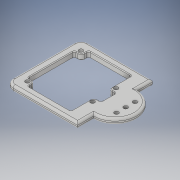
# Autodesk Inventor part: PixyCamMount
Saved by Autodesk Inventor 2018 (Build 220112000, 112)
## iProperties
Created: 2018-09-25
Part Number: PixyCamMount
Material: Generic
Document SubType Name: Modeling
Designer: Jack
Density: 1 g/cm^3
Appearance: Default
Author: Jack
Autodesk Inventor part; units mm, degrees
ref_plane "YZ Plane" through (0, 0, 0) normal (1, 0, 0) x (0, 1, 0)
sketch "Sketch1" plane through (0, 0, 0) normal (0, 1, 0) x (-1, 0, 0)
  line L0 (0, 0) -> (57.15, 0)
  line L1 (63.5, -6.35) -> (63.5, -60.198)
  line L2 (57.15, -66.548) -> (0, -66.548)
  line L3 (12.7, -6.35) -> (50.8, -6.35)
  line L4 (12.7, -6.35) -> (50.8, -6.35) construction
  line L5 (57.15, -12.7) -> (57.15, -53.848)
  line L6 (50.8, -60.198) -> (12.7, -60.198)
  line L7 (12.7, -19.05) -> (12.7, -6.35)
  line L8 (12.7, -47.498) -> (12.7, -60.198)
  line L9 (50.8, -6.35) -> (50.8, -9.652)
  line L10 (53.848, -12.7) -> (57.15, -12.7)
  line L11 (50.8, -60.198) -> (50.8, -56.896)
  line L12 (53.848, -53.848) -> (57.15, -53.848)
  line L13 (12.7, -19.05) -> (12.7, -23.622)
  line L14 (9.652, -26.67) -> (6.35, -26.67)
  line L15 (12.7, -47.498) -> (12.7, -42.926)
  line L16 (9.652, -39.878) -> (6.35, -39.878)
  line L17 (6.35, -39.878) -> (6.35, -26.67)
  arc A0 (50.8, -9.652) -> (53.848, -12.7) centre (53.848, -9.652) ccw
  arc A1 (53.848, -53.848) -> (50.8, -56.896) centre (53.848, -56.896) ccw
  arc A2 (9.652, -26.67) -> (12.7, -23.622) centre (9.652, -23.622) ccw
  arc A3 (12.7, -42.926) -> (9.652, -39.878) centre (9.652, -42.926) ccw
  arc A4 (57.15, -66.548) -> (63.5, -60.198) centre (57.15, -60.198) ccw
  arc A5 (63.5, -6.35) -> (57.15, 0) centre (57.15, -6.35) ccw
  circle A6 centre (9.525, -43.688) radius 1.85
  circle A7 centre (9.525, -22.86) radius 1.85
  circle A8 centre (53.975, -57.023) radius 1.85
  circle A9 centre (53.975, -9.525) radius 1.85
  arc A10 (0, -14.224) -> (0, -52.324) centre (0, -33.274) ccw
  circle A11 centre (-9.525, -41.5229) radius 1.85
  circle A12 centre (-9.525, -33.274) radius 1.85
  circle A13 centre (-9.525, -25.0251) radius 1.85
  line L18 (0, -66.548) -> (0, -52.324)
  line L19 (0, -14.224) -> (0, 0)
  point P0 (63.5, -66.548)
  point P1 (63.5, 0)
  dimension "d0" = 63.5
  dimension "d1" = 66.548
  dimension "d35" = 41.148
  dimension "d36" = 38.1
  dimension "d37" = 13.208
  dimension "d38" = 50.8
  dimension "d39" = 53.848
  dimension "d40" = 3.048
  dimension "d41" = 6.35
  dimension "d81" = 3.7
  dimension "d82" = 3.7
  dimension "d83" = 3.7
  dimension "d84" = 3.7
  dimension "d90" = 3.7
  dimension "d91" = 3.7
  dimension "d92" = 3.7
  constraints: 40 end point, 14 centre point, 14 point on circle, 12 tangent, 10 perpendicular, 4 equal radius, 4 point on line, 4 vertical, 3 horizontal, 3 parallel
  measures "d0" distance of point (63.5, -66.548) L2.end
  measures "d1" distance of point (63.5, 0) point (63.5, -66.548)
  measures "d35" distance of L5.start L5.end
  measures "d36" distance of L3.start L3.end
  measures "d37" distance of L16.end L14.end
  measures "d38" distance between parallel lines of L17 L5
  measures "d39" distance between parallel lines of L6 L3
  measures "d40" radius of A0
  measures "d41" radius of A4
  measures "d81" diameter of A6
  measures "d82" diameter of A7
  measures "d83" diameter of A8
  measures "d84" diameter of A9
  measures "d90" diameter of A11
  measures "d91" diameter of A12
  measures "d92" diameter of A13
ref_plane "Work Plane2" through (0, 5.08, 0) normal (0, 1, 0) x (1, 0, 0)
sketch "Sketch2" plane through (0, 5.08, 0) normal (0, 1, 0) x (1, 0, 0)
  line L0 (-53.4694, 12.7) -> (-55.2474, 12.7)
  line L1 (-50.4214, 12.7) -> (-48.6434, 12.7) construction
  line L2 (-56.7714, 14.224) -> (-56.7714, 52.324)
  line L3 (-55.2474, 53.848) -> (-53.4694, 53.848)
  line L4 (-50.4214, 56.896) -> (-50.4214, 58.674)
  line L5 (-48.8974, 60.198) -> (-13.8454, 60.198)
  line L6 (-12.3214, 58.674) -> (-12.3214, 42.926)
  line L7 (-9.2734, 39.878) -> (-7.4954, 39.878)
  line L8 (-5.9714, 38.354) -> (-5.9714, 28.194)
  line L9 (-7.4954, 26.67) -> (-9.2734, 26.67)
  line L10 (-12.3214, 23.622) -> (-12.3214, 7.874)
  line L11 (-12.3214, 26.67) -> (3.4266, 26.67) construction
  line L12 (-13.8454, 6.35) -> (-48.8974, 6.35)
  line L13 (-50.4214, 7.874) -> (-50.4214, 9.652)
  arc A0 (-50.4214, 9.652) -> (-53.4694, 12.7) centre (-53.4694, 9.652) ccw
  arc A1 (-53.4694, 53.848) -> (-50.4214, 56.896) centre (-53.4694, 56.896) ccw
  arc A2 (-9.2734, 26.67) -> (-12.3214, 23.622) centre (-9.2734, 23.622) ccw
  arc A3 (-12.3214, 42.926) -> (-9.2734, 39.878) centre (-9.2734, 42.926) ccw
  arc A4 (-50.4214, 7.874) -> (-48.8974, 6.35) centre (-48.8974, 7.874) ccw
  arc A5 (-13.8454, 6.35) -> (-12.3214, 7.874) centre (-13.8454, 7.874) ccw
  arc A6 (-12.3214, 58.674) -> (-13.8454, 60.198) centre (-13.8454, 58.674) ccw
  arc A7 (-48.8974, 60.198) -> (-50.4214, 58.674) centre (-48.8974, 58.674) ccw
  arc A8 (-55.2474, 53.848) -> (-56.7714, 52.324) centre (-55.2474, 52.324) ccw
  arc A9 (-56.7714, 14.224) -> (-55.2474, 12.7) centre (-55.2474, 14.224) ccw
  arc A10 (-7.4954, 26.67) -> (-5.9714, 28.194) centre (-7.4954, 28.194) ccw
  arc A11 (-5.9714, 38.354) -> (-7.4954, 39.878) centre (-7.4954, 38.354) ccw
  point P0 (0, 0)
  point P1 (-56.7714, 12.7)
  point P2 (-56.7714, 53.848)
  point P3 (-50.4214, 53.848)
  point P4 (-50.4214, 60.198)
  point P5 (-12.3214, 60.198)
  point P6 (-12.3214, 39.878)
  point P7 (-5.9714, 39.878)
  point P8 (-5.9714, 26.67)
  point P9 (-12.3214, 6.35)
  point P10 (-50.4214, 6.35)
  dimension "d44" = 6.35
  dimension "d45" = 180
  dimension "d46" = 41.148
  dimension "d47" = 90
  dimension "d48" = 6.35
  dimension "d49" = 90
  dimension "d50" = 6.35
  dimension "d51" = 90
  dimension "d52" = 38.1
  dimension "d53" = 90
  dimension "d54" = 20.32
  dimension "d55" = 90
  dimension "d56" = 6.35
  dimension "d57" = 90
  dimension "d58" = 13.208
  dimension "d59" = 90
  dimension "d60" = 6.35
  dimension "d61" = 90
  dimension "d62" = 20.32
  dimension "d63" = 90
  dimension "d64" = 38.1
  dimension "d65" = 90
  dimension "d66" = 3.048
  dimension "d67" = 1.524
  constraints: 28 end point, 24 point on circle, 24 point on line, 24 tangent, 12 centre point, 10 equal radius, 9 perpendicular, 3 horizontal, 2 equal length, 1 vertical
  measures "d44" distance of L1.start point (-56.771, 12.7)
  measures "d45" angle of L0 L1
  measures "d46" distance of point (-56.771, 12.7) point (-56.771, 53.848)
  measures "d47" angle of L0 L2
  measures "d48" distance of point (-56.771, 53.848) point (-50.421, 53.848)
  measures "d49" angle of L2 L3
  measures "d50" distance of point (-50.421, 53.848) point (-50.421, 60.198)
  measures "d51" angle of L4 L3
  measures "d52" distance of point (-50.421, 60.198) point (-12.321, 60.198)
  measures "d53" angle of L4 L5
  measures "d54" distance of point (-12.321, 60.198) point (-12.321, 39.878)
  measures "d55" angle of L5 L6
  measures "d56" distance of point (-12.321, 39.878) point (-5.971, 39.878)
  measures "d57" angle of L7 L6
  measures "d58" distance of point (-5.971, 39.878) point (-5.971, 26.67)
  measures "d59" angle of L7 L8
  measures "d60" distance of point (-5.971, 26.67) L11.start
  measures "d61" angle of L8 L9
  measures "d62" distance of L11.start point (-12.321, 6.35)
  measures "d63" angle of L10 L11
  measures "d64" distance of point (-12.321, 6.35) point (-50.421, 6.35)
  measures "d65" angle of L10 L12
  measures "d66" radius of A0
  measures "d67" radius of A4
ref_plane "Work Plane1" through (0, 0, 0) normal (1, 0, 0) x (0, 0, -1)
extrude "Extrusion6" add sketch "Sketch1" along normal blind 5.08 contours L0 A5 L1 A4 L2 L18 A10 L19 | L3 L9 A0 L10 L5 L12 A1 L11 L6 L8 L15 A3 L16 L17 L14 A2 L13 L7
extrude "Extrusion7" cut sketch "Sketch2" against normal blind 5.08
fillet "Fillet2" radius 0.635 48 edges at (-11.4287, 5.08, -40.7707) (-8.3844, 5.08, -39.878) (-6.4178, 5.08, -39.4316) (-5.9714, 5.08, -33.274) (-6.4178, 5.08, -27.1164) (-8.3844, 5.08, -26.67) (-11.4287, 5.08, -25.7773) (-12.3214, 5.08, -15.748) (-12.7678, 5.08, -6.7964) (-31.3714, 5.08, -6.35) (-49.975, 5.08, -6.7964) (-50.4214, 5.08, -8.763) (-51.3141, 5.08, -11.8073) (-54.3584, 5.08, -12.7) (-56.325, 5.08, -13.1464) (-56.7714, 5.08, -33.274) (-56.325, 5.08, -53.4016) (-54.3584, 5.08, -53.848) (-51.3141, 5.08, -54.7407) (-50.4214, 5.08, -57.785) (-49.975, 5.08, -59.7516) (-31.3714, 5.08, -60.198) (-12.7678, 5.08, -59.7516) (-12.3214, 5.08, -50.8) (-56.325, 0, -13.1464) (-54.3584, 0, -12.7) (-51.3141, 0, -11.8073) (-50.4214, 0, -8.763) (-49.975, 0, -6.7964) (-31.3714, 0, -6.35) (-12.7678, 0, -6.7964) (-12.3214, 0, -15.748) (-11.4287, 0, -25.7773) (-8.3844, 0, -26.67) (-6.4178, 0, -27.1164) (-5.9714, 0, -33.274) (-6.4178, 0, -39.4316) (-8.3844, 0, -39.878) (-11.4287, 0, -40.7707) (-12.3214, 0, -50.8) (-12.7678, 0, -59.7516) (-31.3714, 0, -60.198) (-49.975, 0, -59.7516) (-50.4214, 0, -57.785) (-51.3141, 0, -54.7407) (-54.3584, 0, -53.848) (-56.325, 0, -53.4016) (-56.7714, 0, -33.274)
fillet "Fillet3" radius 1.905 16 edges at (19.05, 5.08, -33.274) (0, 5.08, -59.436) (0, 5.08, -7.112) (-61.6401, 5.08, -1.8599) (-63.5, 5.08, -33.274) (-61.6401, 5.08, -64.6881) (-28.575, 5.08, -66.548) (-28.575, 5.08, 0) (-61.6401, 0, -64.6881) (-28.575, 0, -66.548) (-61.6401, 0, -1.8599) (-28.575, 0, 0) (-63.5, 0, -33.274) (0, 0, -59.436) (19.05, 0, -33.274) (0, 0, -7.112)
body "Solid1"
